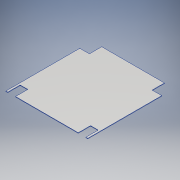
# Autodesk Inventor part: BK-BKT120-BasePlateextruded
Saved by Autodesk Inventor 2017 (Build 210142000, 142)
## iProperties
Created: 2016-09-24
Part Number: BK-BKT120-BasePlateextruded
Material: Aluminum 6061
Document SubType Name: Modeling
Designer: vslabsal
Density: 2.7 g/cm^3
Appearance: Aluminum - Flat
Author: vslabsal
Autodesk Inventor part; units mm, degrees
ref_plane "YZ Plane" through (0, 0, 0) normal (1, 0, 0) x (0, 1, 0)
ref_plane "XZ Plane" through (0, 0, 0) normal (0, 1, 0) x (-1, 0, 0)
ref_plane "XY Plane" through (0, 0, 0) normal (0, 0, 1) x (1, 0, 0)
sketch "Sketch1" plane through (0, 0, 0) normal (0, 0, 1) x (1, 0, 0)
  line L0 (270.51, 284.48) -> (-270.51, -284.48) construction
  line L1 (-270.51, 284.48) -> (270.51, -284.48) construction
  line L2 (-270.51, -284.48) -> (-257.81, -284.48)
  line L3 (-207.01, -284.48) -> (207.01, -284.48)
  line L4 (257.81, -284.48) -> (270.51, -284.48)
  line L5 (270.51, -284.48) -> (270.51, 203.2)
  line L6 (207.005, 284.48) -> (-207.015, 284.48)
  line L7 (-207.015, 206.375) -> (-207.015, 284.48)
  line L8 (-210.185, 203.2) -> (-270.51, 203.2)
  line L9 (-270.51, 203.2) -> (-270.51, -284.48)
  arc A0 (-210.185, 203.2) -> (-207.015, 206.375) centre (-210.19, 206.375) ccw
  line L10 (207.005, 284.48) -> (207.005, 206.375)
  line L11 (270.51, 203.2) -> (210.185, 203.2)
  arc A1 (207.005, 206.375) -> (210.185, 203.2) centre (210.18, 206.375) ccw
  line L12 (-257.81, -284.48) -> (-257.81, -206.375)
  line L13 (-207.01, -284.48) -> (-207.01, -206.375)
  arc A2 (-254.635, -203.2) -> (-257.81, -206.375) centre (-254.635, -206.375) ccw
  arc A3 (-207.01, -206.375) -> (-210.185, -203.2) centre (-210.185, -206.375) ccw
  line L14 (-254.635, -203.2) -> (-210.185, -203.2)
  line L15 (207.01, -284.48) -> (207.01, -206.375)
  line L16 (257.81, -284.48) -> (257.81, -206.375)
  arc A4 (210.185, -203.2) -> (207.01, -206.375) centre (210.185, -206.375) ccw
  arc A5 (257.81, -206.375) -> (254.635, -203.2) centre (254.635, -206.375) ccw
  line L17 (210.185, -203.2) -> (254.635, -203.2)
  point P0 (0, 0)
  point P1 (0, 0)
  dimension "d0" = 541.02
  dimension "d1" = 568.96
  dimension "d2" = 12.7
  dimension "d6" = 414.02
  dimension "d10" = 12.7
  dimension "d11" = 487.68
  dimension "d14" = 414.02
  dimension "d19" = 78.105
  dimension "d20" = 60.325
  dimension "d22" = 78.105
  dimension "d23" = 60.325
  dimension "d26" = 78.105
  dimension "d27" = 78.105
  dimension "d28" = 44.45
  dimension "d29" = 50.8
  dimension "d30" = 78.105
  dimension "d31" = 78.105
  constraints: 36 end point, 18 point on circle, 8 horizontal, 8 vertical, 6 centre point, 2 midpoint, 1 point on line, 1 tangent
  measures "d0" distance of L0.end L1.end
  measures "d1" distance of L1.start L0.end
  measures "d2" distance of L0.end L2.end
  measures "d6" distance of L3.start L3.end
  measures "d10" distance of L4.start L1.end
  measures "d11" distance of L1.end L5.end
  measures "d14" distance of L6.end L6.start
  measures "d19" distance of L7.start L6.end
  measures "d20" distance of L8.start L8.end
  measures "d22" distance of L6.start L10.end
  measures "d23" distance of L5.end L11.end
  measures "d26" distance of L3.start L13.end
  measures "d27" distance of L2.end L12.end
  measures "d28" distance of L14.start L14.end
  measures "d29" distance between parallel lines of L13 L12
  measures "d30" distance of L3.end L15.end
  measures "d31" distance of L4.start L16.end
extrude "Extrusion1" add sketch "Sketch1" along normal blind 3.175
body "Solid1"
